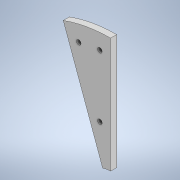
# Autodesk Inventor part: cover2
Saved by Autodesk Inventor 2020.3 (Build 243373000, 373)
## iProperties
Created: 2020-11-01
Part Number: cover2
Material: Generic
Document SubType Name: Modeling
Designer: Martijn
Density: 1 g/cm^3
Appearance: Default
Author: Martijn
Autodesk Inventor part; units mm, degrees
ref_plane "YZ Plane" through (0, 0, 0) normal (1, 0, 0) x (0, 1, 0)
ref_plane "XZ Plane" through (0, 0, 0) normal (0, 1, 0) x (-1, 0, 0)
ref_plane "XY Plane" through (0, 0, 0) normal (0, 0, 1) x (1, 0, 0)
sketch "Sketch1" plane through (0, 0, 0) normal (0, 0, 1) x (1, 0, 0)
  arc A0 (0, 90) -> (77.9423, -45) centre (0, 0) ccw
  line L0 (0, 5) -> (0, 90)
  line L1 (77.9423, -45) -> (4.3301, -2.5)
  line L2 (0, 5) -> (0, 0)
  line L3 (0, 0) -> (4.3301, -2.5)
  line L4 (0, -167.6192) -> (0, 145.1192) projected
  dimension "d0" = 120
  dimension "d2" = 90
  constraints: 8 end point, 3 collinear, 2 coincident, 2 point on circle, 1 centre point
  measures "d0" angle of L1 L0
  measures "d2" radius of A0
extrude "Extrusion1" add sketch "Sketch1" along normal blind 4
sketch "Sketch2" plane through (0, 0, 0) normal (0, 0, -1) x (-1, 0, 0)
  circle A0 centre (20.7055, 77.2741) radius 1.5
  circle A1 centre (6.9459, 39.3923) radius 1.5
  line L0 (0, 0) -> (0, 90) projected
  line L1 (20.7055, 77.2741) -> (0, 0)
  circle A2 centre (6.9725, 79.6956) radius 1.5
  line L2 (6.9725, 79.6956) -> (0, 0)
  line L3 (6.9459, 39.3923) -> (0, 0)
  dimension "d5" = 3
  dimension "d6" = 3
  dimension "d7" = 80
  dimension "d9" = 15
  dimension "d16" = 80
  dimension "d17" = 3
  dimension "d18" = 5
  dimension "d27" = 5
  dimension "d28" = 40
  constraints: 6 end point, 3 centre point
  measures "d5" diameter of A1
  measures "d6" diameter of A0
  measures "d7" distance of L1.start L0.start
  measures "d9" angle of L0 L1
  measures "d16" distance of L2.start L0.start
  measures "d17" diameter of A2
  measures "d18" angle of L0 L2
  measures "d27" angle of L2 L3
  measures "d28" distance of L3.start L0.start
extrude "Extrusion2" cut sketch "Sketch2" against normal blind 10
pattern_circular "Circular Pattern1" count 12 over 220 about axis through (0, 0, 0) along (0, 0, 1) of "Extrusion2"
sketch "Sketch4" plane through (0, 0, 0) normal (0, 0, -1) x (-1, 0, 0)
  circle A0 centre (0, 0) radius 15
  dimension "d29" = 30
  constraints: 1 centre point, 1 coincident
  measures "d29" diameter of A0
extrude "Extrusion4" cut sketch "Sketch4" against normal blind 10
sketch "Sketch5" plane through (0, 0, 4) normal (0, 0, 1) x (1, 0, 0)
  arc A0 (0, 15) -> (12.9904, -7.5) centre (0, 0) ccw projected
  line L0 (0, 0) -> (-30.7818, 84.5723)
  arc A1 (0, 90) -> (77.9423, -45) centre (0, 0) ccw projected
  line L1 (0, 0) -> (77.9423, -45)
  arc A2 (-30.7818, 84.5723) -> (77.9423, -45) centre (0, 0) ccw
  line L2 (0, 15) -> (0, 90) projected
  point P0 (12.9904, -7.5)
  point P1 (-5.1303, 14.0954)
  dimension "d32" = 20
  constraints: 4 end point, 3 point on circle, 1 centre point, 1 coincident
  measures "d32" angle of L2 L0
extrude "Extrusion5" cut sketch "Sketch5" against normal blind 10 contours A0 L1 A1 L0
body "Solid1"
